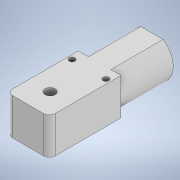
# Autodesk Inventor part: Yellow_Motor
Saved by Autodesk Inventor 2022.2 (Build 262287000, 287)
## iProperties
Created: 2022-06-29
Part Number: Yellow_Motor
Material: Generic
Document SubType Name: Modeling
Designer: ABL
Density: 1 g/cm^3
Appearance: Default
Author: ABL
Autodesk Inventor part; units mm, degrees
ref_plane "YZ Plane" through (0, 0, 0) normal (1, 0, 0) x (0, 1, 0)
ref_plane "XZ Plane" through (0, 0, 0) normal (0, 1, 0) x (-1, 0, 0)
ref_plane "XY Plane" through (0, 0, 0) normal (0, 0, 1) x (1, 0, 0)
sketch "Sketch1" plane through (0, 0, 0) normal (0, 1, 0) x (-1, 0, 0)
  line L0 (0, 0) -> (-22, 0)
  line L1 (-22, 0) -> (-22, -37)
  line L2 (-22, -37) -> (0, -37)
  line L3 (0, -37) -> (0, 0)
  line L4 (-11, -37) -> (-11, 0) construction
  circle A0 centre (-11, -11.4) radius 2.65
  circle A1 centre (-19.75, -31.5) radius 1.5
  circle A2 centre (-2.25, -31.5) radius 1.5
  dimension "gearboxWidth" = 22
  dimension "gearboxLength" = 37
  dimension "shaftDiameter" = 5.3
  dimension "shaftCenterToBottom" = 11.4
  dimension "mountHolesDiameter" = 3
  dimension "mountHolesCenterToCenter" = 17.5
  dimension "mountHolesCenterToEdge" = 5.5
  constraints: 10 end point, 3 centre point, 2 midpoint, 2 parallel, 1 horizontal, 1 perpendicular, 1 point on line, 1 symmetric about line, 1 other
  measures "gearboxWidth" distance of L2.end L1.end
  measures "gearboxLength" distance of L1.end L0.end
  measures "shaftDiameter" diameter of A0
  measures "shaftCenterToBottom" distance of L4.end A0.centre
  measures "mountHolesDiameter" diameter of A1
  measures "mountHolesCenterToCenter" diameter of A1.centre L4
  measures "mountHolesCenterToEdge" distance from line of A1.centre L2
extrude "Extrusion1" add sketch "Sketch1" along normal blind 19
sketch "Sketch2" plane through (22, 0, -37) normal (0, 0, -1) x (-1, 0, 0)
  line L0 (0, 19) -> (22, 19) projected
  line L1 (11, 19) -> (11, 0) construction
  line L2 (0, 0) -> (22, 0) projected
  ellipse E0 centre (11, 9.5) end of major axis (22, 9.5) minor radius 11.1399 (16.7448, 0) -> (16.7448, 19) ccw
  ellipse E1 centre (11, 9.5) end of major axis (22, 9.5) minor radius 11.1399 (5.2552, 19) -> (5.2552, 0) ccw
  line L3 (5.2552, 19) -> (16.7448, 19)
  line L4 (5.2552, 0) -> (16.7448, 0)
  constraints: 6 end point, 4 point on line, 3 midpoint, 1 horizontal, 8 other
extrude "Extrusion2" add sketch "Sketch2" along normal blind 27
fillet "Fillet1" radius 3 2 edges at (0, 9.5, 0) (22, 9.5, 0)
body "Solid1"
